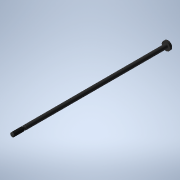
# Autodesk Inventor part: 19182 DSNU-8-100-P---(A---00--0-KS)
Saved by Autodesk Inventor 2021 (Build 250183000, 183)
## iProperties
Created: 2026-04-16
Part Number: 19182 DSNU-8-100-P---(A---00--0-KS)
Material: Generic
Catalog Web Link: www.3dfindit.com
Description: DSNU---(KS)-ISO cylinder
Vendor: FESTO
Document SubType Name: Modeling
Designer: psAdmin
Manufacturer: FESTO
Mass: 1.94536 g
Surface Area: 20.0019 cm^2
Volume: 1.94536 cm^3
Density: 1 g/cm^3
Appearance: PSOLRGB-176-176-176
Category: PARTsolutions
Company: FESTO
Title: 19182 DSNU-8-100-P
Author: Cadenas PARTsolutions
Comments: ISO cylinder
PSOL_IDENT_0: {$CADENAS_DATA/23d-libs/festo/parts/d/dsnu/parts/dsnu_metric_ks.prj},255 {VTYP=3D},{NB=19182 DSNU-8-
PSOL_IDENT_1: 100-P---(A---00--0-KS)},{LINA=19182 DSNU-8-100-P},{NN=DSNU---(KS)},{DATE=03.04.2026 17:15:03},{GEOMD
PSOL_IDENT_2: ATE=26.03.2026 08:56:36},{VERSION=},{LINEID=10},{WBVAR=TNR,HUB,DA,PE,ZD,VS,KA,HE,K2A,K6,K3,K5,K8,KP}
PSOL_IDENT_3: ,{WBNUMERIC=HUB,K2A,K6,K8}  {NB=19182 DSNU-8-100-P---(A---00--0-KS)},{LINA=19182 DSNU-8-100-P},{KT=D
PSOL_IDENT_4: UMMY},{TNR=19182},{TYP=DSNU-8},{DSNU=METRIC},{KDM=8},{HUB=100},{DA=P},{DA1='P'},{PE=A},{ZD=-},{VS=-}
PSOL_IDENT_5: ,{VSALG='-'},{KA=-},{KAALG='-','S2'},{HE=-},{HE1='-','15KE'},{HET=},{K2A=0},{K6=0},{K3=-},{K31='-'},
PSOL_IDENT_6: {K5=-},{K51='-'},{K8=0},{KP=-},{KPALG='-','KP'},{A1=15},{A2=500},{A3=4},{A4=29.0},{AB=12},{AM=12},{B=
PSOL_IDENT_7: 12},{BB=3},{BE=M12x1,25},{BENDM=12.000},{BEKDM=10.466},{BEP=1.250},{BS=3.4},{B1=24},{B2=0},{B3=0},{B
PSOL_IDENT_8: 4=0},{B5=14.0},{B6=6},{B7=0},{CD=4},{D=15},{D1=12},{D2=4},{D3=9.3},{D4=0.0},{D5=10.5},{D6=0},{D7=0},
PSOL_IDENT_9: {EE=M5},{EENDM=5.000},{EEKDM=4.019},{EW=8},{F=18},{FF=M3},{FFNDM=3.000},{FFKDM=2.387},{F1=0},{H=16},
PSOL_IDENT_10: {H1=0},{KK=M4},{KKNDM=4.000},{KKKDM=0.000},{KKP=0.700},{K1=-},{K1NDM=0.000},{K1KDM=0.000},{K2=0.0},{
PSOL_IDENT_11: KV=19},{KW=6},{L=6},{LH=5.0},{LK=7.6},{L1=74},{L2=46},{L3=6.0},{L4=12.0},{L5=10},{L6=28},{L7=16},{L8=
PSOL_IDENT_12: 10.0},{L9=16.0},{L10=53.7},{L11=61.7},{L12=43.6},{L13=78.0},{ST=3.4},{SW=0},{T=0},{WH=16},{X=0.0},{X
PSOL_IDENT_13: C=64},{K1KP=27},{K2KP=M5},{K2KPNDM=5.000},{K3KP=11},{K4KP=13.5},{K5KP=34.5},{K6KP=4.2},{K7KP=12},{K8
PSOL_IDENT_14: KP=19.5},{K9KP=8.0},{K10KP=0.0},{K11KP=0},{K12KP=M5},{K12KPNDM=5.000},{K13KP=29},{ZRSTART=22},{MHL=1
PSOL_IDENT_15: 7.700},{ZRL=26},{C=9.500},{WHX=8.000},{LD1=10.300},{LD2=10.000},{AD1=7.000},{AD2=5.000},{AD3=8.000},
PSOL_IDENT_16: {AD4=6.000},{AD5=0.000},{MH1=6.000},{MH2=2.400},{MH3=8.000},{KP1=16.000},{KP2=9.500},{KP3=7.000},{KP
PSOL_IDENT_17: 4=12.000},{KP5=16.000},{KPC=10.000},{KPF=2.000},{KPG=7.000},{KPH=28.000},{KPJ=11.500},{KPK=10.500},{
PSOL_IDENT_18: KPL=1.500},{KPR3=0.400},{KPR=11.000},{KPS=6.000},{MLD1=25.000},{MLD2=20.000},{MLD3=3.000},{MLL1=8.00
PSOL_IDENT_19: 0},{KL1=35.5},{KKC=3.2},{KKD=1.2},{KKF=0.4},{SWL=0.000},{K3L=0.000},{HUB1=100},{FDTXF31=2.000},{FDTB
PSOL_IDENT_20: 31=2.200},{A5=0},{L01=0},{L02=0},{D01=0},{D01P=0},{D02=0},{R01=0}
NB: 19182 DSNU-8-100-P---(A---00--0-KS)
NN: DSNU---(KS)
NT: ISO cylinder
NBSYN: $TNR. $TYP.-$HUB1.-$DA.---($PE.$ZD.$VS.$KA.$HET.$K2A.$K6.$K3.$K5.$K8.$KP.KS)
LINA: 19182 DSNU-8-100-P
CATALOG: Festo
TNR: 19182
TYP: DSNU-8
DSNU: METRIC
KDM: 8
HUB: 100
DA: P
DA1: 'P'
PE: A
ZD: -
VS: -
KA: -
HE: -
K2A: 0
K6: 0
K3: -
K31: '-'
K5: -
K51: '-'
K8: 0
KP: -
A1: 15
A2: 500
A3: 4
A4: 29
AB: 12
AM: 12
B: 12
BB: 3
BE: M12x1,25
BENDM: 12
BEKDM: 10.466
BEP: 1.25
BS: 3.4
B1: 24
B2: 0
B3: 0
B4: 0
B5: 14
B6: 6
B7: 0
CD: 4
D: 15
D1: 12
D2: 4
D3: 9.3
D4: 0
D5: 10.5
D6: 0
D7: 0
EE: M5
EENDM: 5
EEKDM: 4.019
EW: 8
F: 18
FF: M3
FFNDM: 3
FFKDM: 2.387
F1: 0
H: 16
H1: 0
KK: M4
KKNDM: 4
KKKDM: 0
KKP: 0.7
K1: -
K1NDM: 0
K1KDM: 0
K2: 0
KV: 19
KW: 6
L: 6
LH: 5
LK: 7.6
L3: 6
L4: 12
L5: 10
L6: 28
L7: 16
L8: 10
L9: 16
L13: 78
ST: 3.4
SW: 0
T: 0
X: 0
K1KP: 27
K2KP: M5
K2KPNDM: 5
K3KP: 11
K4KP: 13.5
K5KP: 34.5
K6KP: 4.2
K7KP: 12
K8KP: 19.5
K9KP: 8
K10KP: 0
K11KP: 0
K12KP: M5
K12KPNDM: 5
K13KP: 29
MHL: 17.7
C: 9.5
WHX: 8
LD1: 10.3
LD2: 10
AD1: 7
AD2: 5
AD3: 8
AD4: 6
AD5: 0
MH1: 6
MH2: 2.4
MH3: 8
KP1: 16
KP2: 9.5
KP3: 7
KP4: 12
KP5: 16
KPC: 10
KPF: 2
KPG: 7
KPH: 28
KPJ: 11.5
KPK: 10.5
KPL: 1.5
KPR3: 0.4
KPR: 11
KPS: 6
MLD1: 25
MLD2: 20
MLD3: 3
MLL1: 8
SWL: 0
K3L: 0
FDTXF31: 2
FDTB31: 2.2
SUPPLIER: FESTO
ARTICLENO: 19182 DSNU-8-100-P---(A---00--0-KS)
BOMINFO: 19182 DSNU-8-100-P
CREATOR: CADENAS GmbH
Autodesk Inventor part; units mm, degrees
sketch "Sketch_2" plane through (0, 0, 0) normal (1, 0, 0) x (0, 1, 0)
  line L0 (0, -133.5) -> (0, 4)
  line L1 (0, 4) -> (2, 4)
  line L2 (2, 4) -> (2, -131.5)
  line L3 (2, -131.5) -> (4, -131.5)
  line L4 (4, -131.5) -> (4, -133.5)
  line L5 (4, -133.5) -> (0, -133.5)
  line L6 (0, -133.5) -> (0, 4)
  constraints: 14 end point
revolve "Revolution1" add sketch "Sketch_2" angle 360 about axis through (0, 0, -133.5) along (0, 0, -1)
sketch "Sketch_6" plane through (0, 0, 0) normal (1, 0, 0) x (0, 1, 0)
  line L0 (0, 3) -> (0, 16)
  line L1 (0, 16) -> (1.5705, 16)
  line L2 (1.5705, 16) -> (2, 15.5705)
  line L3 (2, 15.5705) -> (2, 6.299)
  line L4 (2, 6.299) -> (1.6241, 5.2663)
  arc A0 (1.6241, 5.2663) -> (1.6, 5.1295) centre (2, 5.1295) ccw
  line L5 (1.6, 5.1295) -> (1.6, 4.4)
  arc A1 (1.6, 4.4) -> (2, 4) centre (2, 4.4) ccw
  line L6 (2, 4) -> (2, 3)
  line L7 (2, 3) -> (0, 3)
  line L8 (0, 3) -> (0, 16)
  constraints: 18 end point, 4 point on circle, 2 centre point
revolve "Revolution2" add sketch "Sketch_6" angle 360 about axis through (0, 0, 3) along (0, 0, -1)
thread "Thread1" size "M4x0.7" class "6g" standard "ISO Metric profile" full length
ref_plane "FDT_KSAUFSATZ_XY" through (0, 0, 8.2) normal (0, 0, 1) x (-1, 0, 0)
ref_plane "FDT_KSAUFSATZ_YZ" through (0, 0, 8.2) normal (-1, 0, 0) x (0, -1, 0)
ref_plane "FDT_KSAUFSATZ_ZX" through (0, 0, 8.2) normal (0, -1, 0) x (0, 0, 1)
ref_plane "FDT_NUT_XY" through (0, 0, 8.2) normal (0, 0, 1) x (-1, 0, 0)
ref_plane "FDT_NUT_YZ" through (0, 0, 8.2) normal (-1, 0, 0) x (0, -1, 0)
ref_plane "FDT_NUT_ZX" through (0, 0, 8.2) normal (0, -1, 0) x (0, 0, 1)
ref_plane "KS_XY" through (0, 0, 0) normal (0, 0, -1) x (1, 0, 0)
ref_plane "KS_YZ" through (0, 0, 0) normal (1, 0, 0) x (0, -1, 0)
ref_plane "KS_ZX" through (0, 0, 0) normal (0, -1, 0) x (0, 0, -1)
ref_plane "NUT1_XY" through (0, 0, 12) normal (0, 0, 1) x (1, 0, 0)
ref_plane "NUT1_YZ" through (0, 0, 12) normal (1, 0, 0) x (0, 1, 0)
ref_plane "NUT1_ZX" through (0, 0, 12) normal (0, 1, 0) x (0, 0, 1)
body "Solid1"
